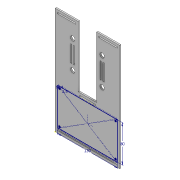
# Autodesk Inventor part: Ushape_top
Saved by Autodesk Inventor 2020 (Build 240168000, 168)
## iProperties
Created: 2021-05-10
Part Number: Ushape_top
Material: Generic
Document SubType Name: Modeling
Designer: Hsu Daniel
Density: 1 g/cm^3
Appearance: Default
Author: Hsu Daniel
Autodesk Inventor part; units mm, degrees
ref_plane "YZ Plane" through (0, 0, 0) normal (1, 0, 0) x (0, 1, 0)
ref_plane "XZ Plane" through (0, 0, 0) normal (0, 1, 0) x (-1, 0, 0)
ref_plane "XY Plane" through (0, 0, 0) normal (0, 0, 1) x (1, 0, 0)
sketch "Sketch1" plane through (0, 0, 0) normal (0, 0, 1) x (1, 0, 0)
  line L0 (0, 0) -> (140, 0)
  line L1 (140, 0) -> (140, 232.6)
  line L2 (140, 232.6) -> (90, 232.6)
  line L3 (90, 232.6) -> (90, 100)
  line L4 (90, 100) -> (50, 100)
  line L5 (50, 100) -> (50, 232.6)
  line L6 (50, 232.6) -> (0, 232.6)
  line L7 (0, 232.6) -> (0, 0)
  line L8 (70, 100) -> (70, 0) construction
  line L9 (30, 232.2963) -> (30, 0) construction
  circle A0 centre (38, 194.6) radius 4.85
  circle A1 centre (38, 134.6) radius 4.85
  circle A2 centre (102, 194.6) radius 4.85
  circle A3 centre (102, 134.6) radius 4.85
  circle A4 centre (30, 194.6) radius 14 construction
  circle A5 centre (30, 134.6) radius 14 construction
  line L10 (5, 227.6) -> (45, 227.6)
  line L11 (45, 227.6) -> (45, 224.6)
  line L12 (45, 224.6) -> (5, 224.6)
  line L13 (5, 224.6) -> (5, 227.6)
  line L14 (53, 95) -> (87, 95)
  line L15 (87, 95) -> (87, 92)
  line L16 (87, 92) -> (53, 92)
  line L17 (53, 92) -> (53, 95)
  line L18 (5, 8) -> (135, 8)
  line L19 (135, 8) -> (135, 5)
  line L20 (135, 5) -> (5, 5)
  line L21 (5, 5) -> (5, 8)
  line L22 (135, 227.6) -> (95, 227.6)
  line L23 (95, 227.6) -> (95, 224.6)
  line L24 (95, 224.6) -> (135, 224.6)
  line L25 (135, 224.6) -> (135, 227.6)
  line L26 (30, 194.6) -> (50, 194.6) construction
  line L27 (30, 134.6) -> (50, 134.6) construction
  circle A6 centre (30, 202.6) radius 4.5
  dimension "d0" = 40
  dimension "d2" = 132.6
  dimension "d3" = 100
  dimension "d4" = 9.7
  dimension "d6" = 60
  dimension "d10" = 28
  dimension "d11" = 8
  dimension "d12" = 8
  dimension "d13" = 5
  dimension "d14" = 5
  dimension "d15" = 5
  dimension "d16" = 3
  dimension "d17" = 3
  dimension "d18" = 5
  dimension "d19" = 3
  dimension "d20" = 3
  dimension "d21" = 5
  dimension "d22" = 5
  dimension "d23" = 5
  dimension "d24" = 3
  dimension "d32" = 9
  dimension "d33" = 8
  dimension "d34" = 30
  dimension "d39" = 20
  dimension "d40" = 50
  constraints: 56 end point, 12 perpendicular, 10 point on line, 7 centre point, 6 parallel, 6 symmetric about line, 4 horizontal, 2 equal radius, 2 midpoint, 1 collinear, 2 other
  measures "d0" distance between parallel lines of L8 L9
  measures "d2" distance of L4.end L5.end
  measures "d3" distance of L8.start L8.end
  measures "d4" diameter of A0
  measures "d6" distance of A0.centre A1.centre
  measures "d10" diameter of A4
  measures "d11" distance of A0.centre L26.start
  measures "d12" distance of A1.centre L27.start
  measures "d13" distance between parallel lines of L6 L10
  measures "d14" distance between parallel lines of L5 L11
  measures "d15" distance between parallel lines of L7 L13
  measures "d16" distance of L12.end L10.start
  measures "d17" distance of L16.end L14.start
  measures "d18" distance between parallel lines of L4 L14
  measures "d19" distance between parallel lines of L3 L15
  measures "d20" distance between parallel lines of L5 L17
  measures "d21" distance between parallel lines of L0 L20
  measures "d22" distance between parallel lines of L7 L21
  measures "d23" distance between parallel lines of L1 L19
  measures "d24" distance of L18.end L19.end
  measures "d32" diameter of A6
  measures "d33" distance of L26.start A6.centre
  measures "d34" distance from line of L6 A6.centre
  measures "d39" distance between parallel lines of L5 L9
  measures "d40" distance between parallel lines of L5 L7
extrude "Extrusion2" add sketch "Sketch1" along normal blind 3 contours L7 L6 L5 L4 L3 L2 L1 L0 | A6
sketch "Sketch2" plane through (0, 0, 3) normal (0, 0, 1) x (1, 0, 0)
  circle A0 centre (38, 194.6) radius 4.85 construction
  line L0 (50, 232.6) -> (0, 232.6) construction
  line L1 (50, 232.6) -> (0, 232.6) construction
  line L2 (36.25, 182.6) -> (33.41, 182.6)
  line L3 (33.41, 182.6) -> (33.41, 146.6)
  line L4 (33.41, 146.6) -> (36.25, 146.6)
  line L5 (36.25, 146.6) -> (36.25, 182.6)
  line L6 (90, 100) -> (50, 100) construction
  line L7 (70, 100) -> (70, 0) construction
  line L8 (39.75, 146.6) -> (42.59, 146.6)
  line L9 (42.59, 146.6) -> (42.59, 182.6)
  line L10 (42.59, 182.6) -> (39.75, 182.6)
  line L11 (39.75, 182.6) -> (39.75, 146.6)
  line L12 (103.75, 182.6) -> (106.59, 182.6)
  line L13 (106.59, 182.6) -> (106.59, 146.6)
  line L14 (106.59, 146.6) -> (103.75, 146.6)
  line L15 (103.75, 146.6) -> (103.75, 182.6)
  line L16 (100.25, 146.6) -> (97.41, 146.6)
  line L17 (97.41, 146.6) -> (97.41, 182.6)
  line L18 (97.41, 182.6) -> (100.25, 182.6)
  line L19 (100.25, 182.6) -> (100.25, 146.6)
  line L20 (33.41, 164.6) -> (7.5179, 164.6)
  circle A1 centre (38, 134.6) radius 4.85 construction
  line L21 (38, 134.6) -> (38, 194.6)
  line L22 (38, 164.6) -> (28.9281, 164.6)
  point P0 (0, 0)
  dimension "d28" = 2.84
  dimension "d31" = 36
  dimension "d35" = 1.75
  dimension "d36" = 3.5
  constraints: 40 end point, 8 symmetric about line, 4 horizontal, 3 collinear, 3 midpoint, 3 parallel, 3 vertical, 1 perpendicular
  measures "d28" distance of L2.start L2.end
  measures "d31" distance of L2.end L3.end
  measures "d35" distance between parallel lines of L5 L21
  measures "d36" distance between parallel lines of L11 L5
extrude "Extrusion3" cut sketch "Sketch2" against normal blind 3
sketch "Sketch3" plane through (0, 0, 3) normal (0, 0, 1) x (1, 0, 0)
  line L0 (5, 90) -> (135, 90)
  line L1 (135, 90) -> (135, 10)
  line L2 (135, 10) -> (5, 10)
  line L3 (5, 10) -> (5, 90)
  line L4 (5, 8) -> (135, 8) construction
  line L5 (5, 8) -> (135, 8) construction
  line L6 (135, 8) -> (135, 92) construction
  line L7 (135, 92) -> (5, 92) construction
  line L8 (5, 92) -> (5, 8) construction
  line L9 (87, 92) -> (53, 92) construction
  line L10 (135, 8) -> (135, 5) construction
  line L11 (5, 92) -> (135, 8) construction
  line L12 (5, 8) -> (135, 92) construction
  line L13 (5, 90) -> (135, 10) construction
  line L14 (5, 10) -> (135, 90) construction
  circle A0 centre (9, 86) radius 1.75
  line L15 (70, 50) -> (70, 68.0363) construction
  line L16 (70, 50) -> (82.7907, 50) construction
  circle A1 centre (131, 86) radius 1.75
  circle A2 centre (9, 14) radius 1.75
  circle A3 centre (131, 14) radius 1.75
  point P0 (0, 0)
  dimension "d37" = 130
  dimension "d38" = 80
  dimension "d41" = 3.5
  dimension "d42" = 4
  dimension "d43" = 4
  constraints: 28 end point, 4 centre point, 4 parallel, 3 horizontal, 3 symmetric about line, 2 collinear, 2 midpoint, 2 perpendicular, 1 vertical, 3 other
  measures "d37" distance of L1.end L2.end
  measures "d38" distance of L0.end L1.end
  measures "d41" diameter of A0
  measures "d42" distance from line of L3 A0.centre
  measures "d43" distance from line of L0 A0.centre
extrude "Extrusion4" cut sketch "Sketch3" against normal blind 10 contours A0 | A1 | A2 | A3
equation "\"d0\" = 0.5 * marshdistance"
equation "\"d2\" = sidewallL"
equation "\"d3\" = Uthick"
equation "\"d6\" = marshmarshD"
equation "\"d34\" = marshedgeD"
equation "\"d39\" = 0.5 * Utip"
equation "\"d35\" = 0.5 * stickL"
equation "\"d36\" = stickL"
equation "\"d43\" = d42"
equation "\"thick\" = 0.5"
equation "\"lrlr\" = 19"
equation "\"lrmid\" = 19.9"
equation "\"lrdepth\" = 3.3"
equation "\"mlr\" = 16.6"
equation "\"mmid\" = 24.7"
equation "\"mdepth\" = 4.5"
equation "\"lrltotal\" = 126.6"
equation "\"mltotal\" = 126.6"
equation "\"lrbetween\" = 52.1"
equation "\"mbetween\" = 49.5"
equation "\"toler\" = 1"
equation "\"tight\" = 0.08"
equation "\"stuckw\" = 6"
equation "\"sidewallL\" = 132.6"
equation "\"heaterH\" = 117.3"
equation "\"Uthick\" = 100"
equation "\"marshmarshD\" = 60"
equation "\"marshedgeD\" = 30"
equation "\"stickL\" = 3.5"
equation "\"wireH\" = 25"
equation "\"marshdistance\" = 80"
equation "\"Utip\" = 40"
body "Solid2"
